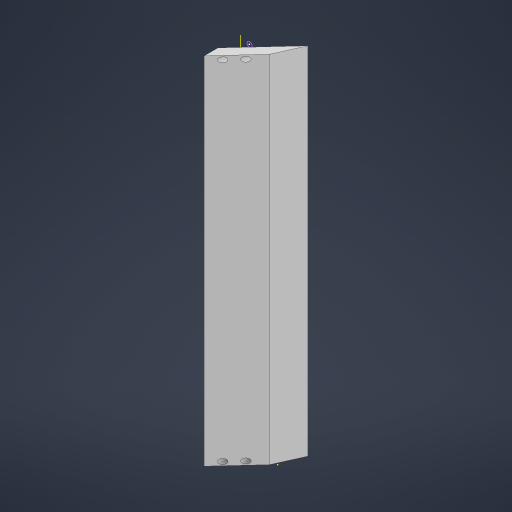
# Autodesk Inventor part: blade
Saved by Autodesk Inventor 2024.3 (Build 283343000, 343)
## iProperties
Created: 2025-05-27
Part Number: blade
Material: Generic
Document SubType Name: Modeling
Designer: Akbar Syihabuddin
Density: 1 g/cm^3
Appearance: Default
Author: Akbar Syihabuddin
Autodesk Inventor part; units mm, degrees
ref_plane "YZ Plane" through (0, 0, 0) normal (1, 0, 0) x (0, 1, 0)
ref_plane "XZ Plane" through (0, 0, 0) normal (0, 1, 0) x (-1, 0, 0)
ref_plane "XY Plane" through (0, 0, 0) normal (0, 0, 1) x (1, 0, 0)
sketch "Sketch1" plane through (0, 0, 0) normal (0, 1, 0) x (-1, 0, 0)
  line L0 (20.0075, 12.0668) -> (-3.1128, -12.9332)
  line L1 (-3.1128, -12.9332) -> (20.0075, 12.0668)
  line L2 (-3.1128, -17.9332) -> (-3.1128, -12.9332)
  line L3 (-3.1128, -17.9332) -> (-14.7232, -17.9332)
  line L4 (-3.1128, -17.9332) -> (-3.1128, -12.9332)
  line L5 (-3.1128, -17.9332) -> (-8.918, -17.9332)
  arc A0 (-14.7232, -17.9332) -> (-3.1128, -12.9332) centre (-21.6099, 14.0384) ccw
  line L6 (-14.7232, -17.9332) -> (20.7671, -17.9332)
  line L7 (20.0075, 12.0668) -> (20.0075, -17.9332)
  line L8 (20.0075, 12.0668) -> (20.0075, 17.0668)
  line L9 (16.3366, 15.4617) -> (-8.1128, -10.9755)
  line L10 (16.3366, 15.4617) -> (20.0075, 19.431)
  line L11 (20.0075, 19.431) -> (20.0075, 15.7489)
  line L12 (-14.7232, -17.9332) -> (-8.1128, -10.9755)
  point P0 (0, 0)
  dimension "d0" = 5
  dimension "d1" = 5
  constraints: 26 end point, 4 point on line, 2 collinear, 2 point on circle, 1 centre point, 1 midpoint, 1 perpendicular
  measures "d0" distance of L0.start L8.end
  measures "d1" distance between parallel lines of L0 L9
extrude "Extrusion1" add sketch "Sketch1" along normal blind 186.69 contours L0 A0 L12 L9 L10 L11 L8
sketch "Sketch2" plane through (0, 0, 0) normal (0, -1, 0) x (1, 0, 0)
  line L0 (3.1128, -12.9332) -> (-20.0075, 12.0668) projected
  line L1 (-20.0075, 12.0668) -> (-16.3304, 12.0668)
  line L2 (-16.3304, 12.0668) -> (-16.3304, -0.4332)
  line L3 (-16.3304, -0.4332) -> (-20.0075, -0.4332)
  line L4 (-20.0075, -0.4332) -> (-20.0075, 12.0668)
  circle A0 centre (-18.1689, 1.5735) radius 1.35
  circle A1 centre (-18.1689, 5.8168) radius 1.35
  point P0 (0, 0)
  point P1 (-16.3304, 8.0908)
  dimension "d4" = 2.7
  dimension "d5" = 2.7
  constraints: 8 end point, 2 centre point, 2 parallel, 1 horizontal, 1 perpendicular
  measures "d4" diameter of A0
  measures "d5" diameter of A1
extrude "Extrusion2" add sketch "Sketch2" along normal blind 3 contours L2 L3 L4 L0
sketch "Sketch3" plane through (0, 0, 0) normal (0, -1, 0) x (1, 0, 0)
  line L0 (-20.0075, 12.0668) -> (-20.0075, 19.431) projected
  line L1 (3.1128, -12.9332) -> (-20.0075, 12.0668) projected
  line L2 (-20.0075, 19.431) -> (-20.0075, 12.0668)
  line L3 (-20.0075, 12.0668) -> (3.1128, -12.9332)
  arc A0 (3.1128, -12.9332) -> (14.7232, -17.9332) centre (21.6099, 14.0384) ccw projected
  arc A1 (3.1128, -12.9332) -> (14.6054, -17.9076) centre (21.6099, 14.0384) ccw
  line L4 (8.1128, -10.9755) -> (14.7232, -17.9332) projected
  line L5 (8.1128, -10.9755) -> (14.7232, -17.9332)
  line L6 (-20.0075, 19.431) -> (8.1128, -10.9755)
  point P0 (0, 0)
  constraints: 8 end point, 3 point on circle, 2 collinear, 1 centre point, 1 vertical
extrude "Extrusion3" add sketch "Sketch3" along normal blind 3
sketch "Sketch4" plane through (0, 186.69, 0) normal (0, 1, 0) x (1, 0, 0)
  circle A0 centre (-18.1689, -5.8168) radius 1.35 projected
  circle A1 centre (-18.1689, -1.5735) radius 1.35 projected
  line L0 (-20.0075, -19.431) -> (-20.0075, 0.4332) projected
  line L1 (-20.0075, 0.4332) -> (-16.3304, 0.4332) projected
  line L2 (-16.3304, 0.4332) -> (-16.3304, -8.0908) projected
  line L3 (8.1128, 10.9755) -> (14.7232, 17.9332) projected
  line L4 (14.7232, 17.9332) -> (8.1128, 10.9755)
  line L5 (-20.0075, -19.431) -> (8.1128, 10.9755) projected
  line L6 (8.1128, 10.9755) -> (-20.0075, -19.431)
  line L7 (-20.0075, -19.431) -> (-20.0075, 0.4332)
  line L8 (-20.0075, 0.4332) -> (-16.3304, 0.4332) projected
  line L9 (-20.0075, 0.4332) -> (-16.3304, 0.4332)
  line L10 (-16.3304, 0.4332) -> (-16.3304, -8.0908)
  line L11 (3.1128, 12.9332) -> (-20.0075, -12.0668) projected
  line L12 (-16.3304, -8.0908) -> (3.1128, 12.9332)
  arc A2 (14.7232, 17.9332) -> (3.1128, 12.9332) centre (21.6099, -14.0384) ccw
  arc A3 (-20.0075, -12.0668) -> (-20.0075, -10.5639) centre (-20.8201, -11.3154) ccw
  line L13 (-16.3304, 0.4332) -> (-20.0075, 0.4332)
  point P0 (0, 0)
  constraints: 14 end point, 6 collinear, 4 point on circle, 2 centre point, 1 perpendicular, 1 point on line, 1 tangent
extrude "Extrusion4" add sketch "Sketch4" along normal blind 3
sketch "Sketch5" plane through (0, 189.69, 0) normal (0, 1, 0) x (1, 0, 0)
  line L0 (-16.3304, -8.0908) -> (3.1128, 12.9332) projected
  line L1 (3.1128, 12.9332) -> (3.1128, 4.2571)
  line L2 (3.1128, 4.2571) -> (16.783, 4.2571)
  line L3 (16.783, 4.2571) -> (16.783, 22.684)
  line L4 (16.783, 22.684) -> (3.1128, 22.684)
  line L5 (3.1128, 22.684) -> (3.1128, 12.9332)
  point P0 (0, 0)
  constraints: 10 end point, 4 perpendicular, 1 point on line, 1 vertical
extrude "Extrusion5" cut sketch "Sketch5" against normal blind 200
sketch "Sketch6" plane through (0, 189.69, 0) normal (0, 1, 0) x (1, 0, 0)
  line L0 (3.1128, 12.9332) -> (-16.3304, -8.0908) projected
  line L1 (3.1128, 12.9332) -> (-3.2785, -1.3419)
  line L2 (-20.0075, -19.431) -> (3.1128, 5.569) projected
  line L3 (3.1128, 5.569) -> (3.1128, 12.9332) projected
  line L4 (3.1128, 5.569) -> (-3.2785, -1.3419)
  line L5 (3.1128, 5.569) -> (3.1128, 12.9332)
  point P0 (0, 0)
  constraints: 6 end point, 1 collinear, 1 point on line
extrude "Extrusion6" cut sketch "Sketch6" against normal blind 200
sketch "Sketch7" plane through (0, -3, 0) normal (0, -1, 0) x (1, 0, 0)
  line L0 (-16.3304, 8.0908) -> (-16.3304, -0.4332) projected
  line L1 (-16.3304, 8.0908) -> (-20.0075, 12.0668) projected
  line L2 (-16.3304, 8.0908) -> (-20.0075, 12.0668)
  line L3 (-20.0075, -0.4332) -> (-20.0075, 19.431) projected
  line L4 (-20.0075, 12.0668) -> (-20.0075, -0.4332)
  line L5 (-16.3304, -0.4332) -> (-20.0075, -0.4332) projected
  line L6 (-20.0075, -0.4332) -> (-16.3304, -0.4332)
  line L7 (-16.3304, -0.4332) -> (-16.3304, 8.0908)
  point P0 (0, 0)
  constraints: 8 end point, 3 collinear, 1 perpendicular
extrude "Extrusion7" cut sketch "Sketch7" against normal blind 222
sketch "Sketch8" plane through (-20.0075, -3, 19.431) normal (0.7341688, 0, 0.678967) x (0.678967, 0, -0.7341688)
  line L0 (0, 0) -> (0, 192.69) projected
  line L1 (0, 192.69) -> (0, 2)
  line L2 (0, 2) -> (41.2163, 2)
  line L3 (41.2163, 2) -> (41.2163, -1.239)
  line L4 (41.2163, -1.239) -> (0, -1.239)
  line L5 (0, -1.239) -> (0, 2)
  point P0 (27.85, 3)
  dimension "d18" = 190.69
  constraints: 10 end point, 2 parallel, 1 horizontal, 1 perpendicular, 1 point on line
  measures "d18" distance of L0.end L1.end
extrude "Extrusion8" cut sketch "Sketch8" against normal blind 222
sketch "Sketch9" plane through (0, 0, 0) normal (0, 0, 1) x (1, 0, 0)
  circle A0 centre (-15.245, 1.0241) radius 1.35
  line L0 (-20.0075, -1) -> (-20.0075, 189.69) projected
  line L1 (-20.0075, 94.345) -> (7.4426, 94.345)
  circle A1 centre (-9.2868, 1.0241) radius 1.35
  circle A2 centre (-15.245, 187.6659) radius 1.35
  circle A3 centre (-9.2868, 187.6659) radius 1.35
  point P0 (0, 0)
  dimension "d21" = 2.7
  dimension "d22" = 2.7
  constraints: 4 centre point, 2 end point, 2 symmetric about line, 1 horizontal, 1 midpoint, 2 other
  measures "d21" diameter of A0
  measures "d22" diameter of A1
extrude "Extrusion9" cut sketch "Sketch9" along normal mid plane 222
sketch "Sketch10" plane through (0, 0, 0) normal (0, 0, 1) x (1, 0, 0)
  circle A0 centre (-15.245, 1.0241) radius 1.35 projected
  circle A1 centre (-15.245, 1.0241) radius 1.35
  circle A2 centre (-9.2868, 1.0241) radius 1.35 projected
  circle A3 centre (-9.2868, 1.0241) radius 1.35
  circle A4 centre (-15.245, 187.6659) radius 1.35 projected
  circle A5 centre (-15.245, 187.6659) radius 1.35
  circle A6 centre (-9.2868, 187.6659) radius 1.35 projected
  circle A7 centre (-9.2868, 187.6659) radius 1.35
  line L0 (-16.595, 1.0241) -> (-20.0075, 1.0241)
  line L1 (-20.0075, -1) -> (-20.0075, 189.69) projected
  line L2 (-20.0075, 1.0241) -> (-20.0075, -1)
  line L3 (-20.0075, -1) -> (-3.2785, -1) projected
  line L4 (-20.0075, -1) -> (-3.2785, -1)
  point P0 (0, 0)
  constraints: 6 end point, 4 coincident, 3 centre point, 2 horizontal, 1 collinear, 1 horizontal alignment, 1 point on line, 2 other
body "Solid1"
